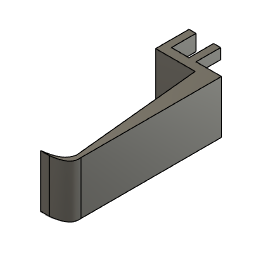
gripper_big (Autodesk Fusion 360 design; units mm, degrees)
Autodesk Fusion 360 part; units mm, degrees
sketch "Sketch1" plane through (0, 0, 0) normal (0, 1, 0) x (1, 0, 0)
  line L0 (-25, 0) -> (-25, 5)
  line L1 (-25, 5) -> (-25, 19)
  line L2 (-25, 19) -> (-21, 19)
  line L3 (-21, 19) -> (-21, 5)
  line L4 (-21, 5) -> (-11, 5)
  line L5 (-11, 5) -> (-11, 19)
  line L6 (-11, 19) -> (-7, 19)
  line L7 (-7, 19) -> (-7, 5)
  line L8 (-7, 5) -> (-2.5, 5)
  line L9 (-2.5, 5) -> (7.5, 5)
  line L10 (7.5, 5) -> (7.5, 0)
  line L11 (-25, 0) -> (-2.5, 0)
  line L12 (7.5, 0) -> (7.5, -5)
  line L13 (-7.4852, -82.9997) -> (-2.5, -83)
  spline S0 degree 5 poles (-7.4852, -82.9997) (-7.0499, -82.9476) (-6.1946, -82.8346) (-4.9577, -82.6382) (-3.4023, -82.3219) (-1.6257, -81.829) (-0.0341, -81.2286) (1.3528, -80.509) (2.5178, -79.6605) (3.4572, -78.6808) (4.1826, -77.5767) (4.6031, -76.6004) (4.8339, -75.819) (4.9508, -75.2766) (5, -75) knots 0 0 0 0 0 0 0.1 0.2 0.3 0.4 0.5 0.6 0.7 0.8 0.9 1 1 1 1 1 1
  line L14 (-2.5, 0) -> (5, -75)
  line L15 (5, -75) -> (7.5, -75)
  line L16 (7.5, -5) -> (7.5, -75)
  spline S1 degree 5 poles (-2.5, -83) (-2.0851, -82.9482) (-1.2732, -82.8357) (-0.1087, -82.64) (1.3356, -82.3244) (2.947, -81.8324) (4.3443, -81.2324) (5.5048, -80.5132) (6.4084, -79.6647) (7.0507, -78.6846) (7.4451, -77.5796) (7.5755, -76.6023) (7.5752, -75.8201) (7.5322, -75.277) (7.5, -75) knots 0 0 0 0 0 0 0.1 0.2 0.3 0.4 0.5 0.6 0.7 0.8 0.9 1 1 1 1 1 1
  point P0 (2, -80)
  point P1 (6, -80)
  constraint perpendicular L15 L16
extrude "Extrude1" add sketch "Sketch1" along normal blind 30
sketch "Sketch2" plane through (-25, 0, 0) normal (-1, 0, 0) x (0, 0, 1)
  line L0 (-19, 0) -> (0, 0)
  line L1 (0, 0) -> (0, 30)
  line L2 (0, 30) -> (-19, 30)
  line L3 (-19, 30) -> (-19, 0)
  line L4 (0, 30) -> (-9, 30)
  line L5 (-9, 0) -> (0, 0)
  line L6 (0, 0) -> (0, 30)
  line L7 (-9, 30) -> (-19, 30)
  line L8 (-19, 30) -> (-19, 21)
  line L9 (-19, 21) -> (-9, 21)
  line L10 (-9, 0) -> (-19, 0)
  line L11 (-19, 0) -> (-19, 9)
  line L12 (-19, 9) -> (-9, 9)
  line L13 (-9, 21) -> (-19, 21)
  line L14 (-19, 21) -> (-19, 9)
  line L15 (-19, 9) -> (-9, 9)
  line L16 (-9, 9) -> (-9, 21)
  constraint horizontal L4
  constraint horizontal L5
  constraint vertical L6
  constraint coincident L1.end L2.start
  constraint horizontal L7
  constraint vertical L8
  constraint horizontal L9
  constraint horizontal L10
  constraint vertical L11
  constraint horizontal L12
  constraint horizontal L13
  constraint vertical L14
  constraint horizontal L15
  constraint vertical L16
extrude "Extrude2" cut sketch "Sketch2" against normal blind 4 contours L3 L9 L12 L13 L14 L15 L16
sketch "Sketch3" plane through (-7, 0, 0) normal (1, 0, 0) x (0, 0, -1)
  line L0 (5, 0) -> (19, 0)
  line L1 (19, 0) -> (19, 30)
  line L2 (19, 30) -> (5, 30)
  line L3 (5, 30) -> (5, 0)
  line L4 (5, 0) -> (19, 0)
  line L5 (19, 0) -> (19, 6)
  line L6 (19, 6) -> (5, 6)
  line L7 (5, 6) -> (5, 0)
  line L8 (5, 30) -> (19, 30)
  line L9 (19, 30) -> (19, 24)
  line L10 (19, 24) -> (5, 24)
  line L11 (5, 24) -> (5, 30)
  dimension "d29" = 6
  dimension "d30" = 6
  constraint horizontal L4
  constraint vertical L5
  constraint horizontal L6
  constraint vertical L7
  constraint coincident L0.start L3.end
  constraint horizontal L8
  constraint vertical L9
  constraint horizontal L10
  constraint vertical L11
  constraint coincident L2.end L3.start
  measures "d29" distance of L0.start L6.end
  measures "d30" distance of L2.end L10.end
extrude "Extrude3" cut sketch "Sketch3" against normal blind 4 contours L1 L3 L6 L10
